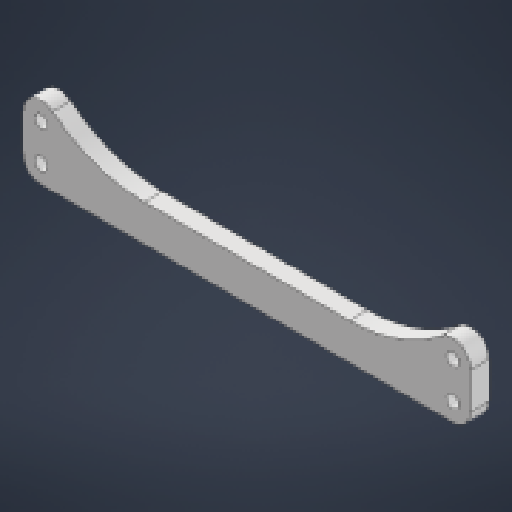
# Autodesk Inventor part: parkbar
Saved by Autodesk Inventor 2025.2 (Build 292293000, 293)
## iProperties
Created: 2025-12-10
Part Number: parkbar
Material: Generic
Document SubType Name: Modeling
Designer: cloudy
Density: 1 g/cm^3
Appearance: Smooth - Dark Gray
Author: cloudy
Autodesk Inventor part; units mm, degrees
ref_plane "YZ Plane" through (0, 0, 0) normal (1, 0, 0) x (0, 1, 0)
ref_plane "XZ Plane" through (0, 0, 0) normal (0, 1, 0) x (-1, 0, 0)
ref_plane "XY Plane" through (0, 0, 0) normal (0, 0, 1) x (1, 0, 0)
sketch "Sketch1" plane through (0, 0, 0) normal (0, 0, 1) x (1, 0, 0)
  circle A0 centre (12.7, -31.75) radius 2.1844 projected
  circle A1 centre (-130.175, -31.75) radius 2.1844 projected
  circle A2 centre (-130.175, -19.05) radius 2.1844 projected
  circle A3 centre (12.7, -19.05) radius 2.1844 projected
  line L0 (12.7, -38.1) -> (-130.175, -38.1)
  line L1 (-136.525, -31.75) -> (-136.525, -19.05)
  line L2 (19.05, -19.05) -> (19.05, -31.75)
  arc A4 (-126.1838, -14.1111) -> (-136.525, -19.05) centre (-130.175, -19.05) ccw
  arc A5 (19.05, -19.05) -> (8.7088, -14.1111) centre (12.7, -19.05) ccw
  arc A6 (-23.221, -25.4) -> (8.7088, -14.1111) centre (-23.221, 25.4) ccw
  arc A7 (-126.1838, -14.1111) -> (-94.254, -25.4) centre (-94.254, 25.4) ccw
  arc A8 (12.7, -38.1) -> (19.05, -31.75) centre (12.7, -31.75) ccw
  arc A9 (-136.525, -31.75) -> (-130.175, -38.1) centre (-130.175, -31.75) ccw
  line L3 (-94.254, -25.4) -> (-23.221, -25.4)
  point P0 (0, 0)
  dimension "d0" = 12.7
  dimension "d1" = 6.35
  dimension "d2" = 6.35
  dimension "d3" = 12.7
  dimension "d4" = 50.8
  dimension "d6" = 6.35
  constraints: 12 point on circle, 10 tangent, 8 end point, 6 centre point, 2 coincident, 2 equal radius, 2 parallel, 1 horizontal, 1 perpendicular
  measures "d0" diameter of A4
  measures "d1" distance from line of L0 A1.centre
  measures "d2" distance from line of A0.centre L2
  measures "d3" diameter of A5
  measures "d4" radius of A6
  measures "d6" radius of A8
extrude "Extrusion1" add sketch "Sketch1" along normal blind 6.35
body "Solid1"
